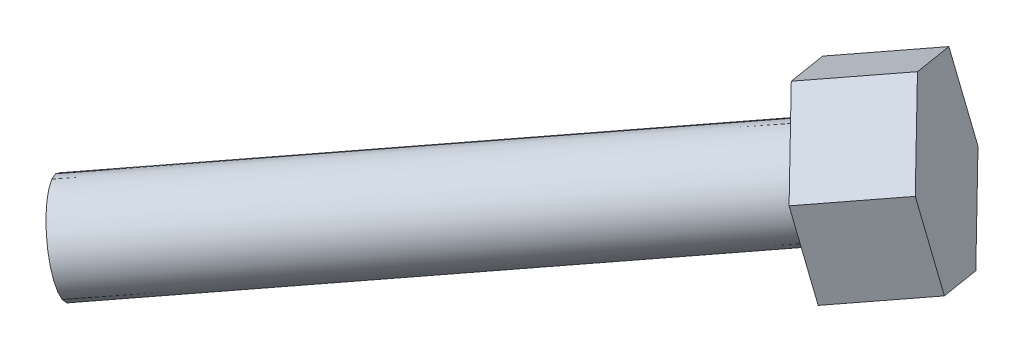
# Autodesk Inventor part: bolt
Saved by Autodesk Inventor 2016 (Build 200138000, 138)
## iProperties
Created: 2016-03-19
Part Number: bolt
Material: Generic
Document SubType Name: Modeling
Designer: gus
Density: 1 g/cm^3
Appearance: Default
Author: gus
Autodesk Inventor part; units mm, degrees
ref_plane "YZ Plane" through (0, 0, 0) normal (1, 0, 0) x (0, 1, 0)
ref_plane "XZ Plane" through (0, 0, 0) normal (0, 1, 0) x (-1, 0, 0)
ref_plane "XY Plane" through (0, 0, 0) normal (0, 0, 1) x (1, 0, 0)
ref_plane "Work Plane1" through (444.1661, 209.2043, 315.1677) normal (0.7992, 0.2064, -0.5645) x (-0.5917, 0.1054, -0.7992)
sketch "Sketch1" plane through (444.1661, 209.2043, 315.1677) normal (0.7992, 0.2064, -0.5645) x (-0.5917, 0.1054, -0.7992)
  line L0 (0, 6.4158) -> (5.5562, 3.2079)
  line L1 (5.5562, 3.2079) -> (5.5562, -3.2079)
  line L2 (5.5562, -3.2079) -> (0, -6.4158)
  line L3 (0, -6.4158) -> (-5.5562, -3.2079)
  line L4 (-5.5562, -3.2079) -> (-5.5562, 3.2079)
  line L5 (-5.5562, 3.2079) -> (0, 6.4158)
  point P0 (492.659, -221.7278)
  point P1 (0, 0)
  point P2 (5.5563, 0)
  dimension "d0" = 11.1125
  constraints: 12 end point, 1 midpoint, 1 vertical, 13 other
  measures "d0" distance between parallel lines of L4 L1
extrude "Extrusion1" add sketch "Sketch1" along normal blind 6.35
sketch "Sketch2" plane through (444.1661, 209.2043, 315.1677) normal (-0.7992, -0.2064, 0.5645) x (0.5917, -0.1054, 0.7992)
  circle A0 centre (0, 0) radius 3.175
  line L0 (-5.5562, 3.2079) -> (-5.5562, -3.2079) projected
  line L1 (0, 6.4158) -> (-5.5562, 3.2079) projected
  point P0 (-492.659, -221.7278)
  dimension "d3" = 6.35
  dimension "d4" = 5.5563
  dimension "d5" = 5.5563
  constraints: 1 centre point
  measures "d3" diameter of A0
  measures "d4" distance from line of L0 A0.centre
  measures "d5" distance from line of L1 A0.centre
extrude "Extrusion2" add sketch "Sketch2" along normal blind 38.1
body "Solid1"
